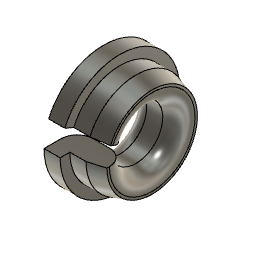
Cable Clamp (Autodesk Fusion 360 design; units mm, degrees)
Autodesk Fusion 360 part; units mm, degrees
note: some values were not read from the file. Set by a fixed rule: which sketch regions a step uses.
sketch "Sketch1" plane through (-35, 0, 0) normal (-1, 0, 0) x (0, -1, 0)
  circle A0 centre (-0.0027, 6.5006) radius 3
  spline S0 degree 3 poles (-2.3623, 9.8149) (-2.8292, 9.5488) (-3.2386, 9.1926) (-3.9138, 8.3291) (-4.1668, 7.8254) (-4.4751, 6.73) (-4.5197, 6.1469) (-4.3843, 4.9751) (-4.1979, 4.3986) (-3.7061, 3.5075) (-3.4567, 3.1707) (-2.8705, 2.5635) (-2.5345, 2.2973) (-2.1684, 2.078) knots 0 0 0 0 0.161221 0.161221 0.328565 0.328565 0.502029 0.502029 0.68161 0.68161 0.806401 0.806401 0.933976 0.933976 0.933976 0.933976
  arc A1 (-2.1684, 2.078) -> (2.1684, 2.078) centre (0, 6.5) ccw
  spline S1 degree 3 poles (2.1684, 2.078) (2.708, 2.4013) (3.1804, 2.8252) (3.9206, 3.816) (4.1875, 4.3686) (4.4856, 5.5258) (4.5215, 6.1173) (4.3635, 7.2597) (4.1789, 7.8006) (3.7084, 8.6093) (3.4817, 8.9033) (2.9632, 9.4172) (2.6753, 9.6365) (2.3623, 9.8149) knots 0 0 0 0 0.188714 0.188714 0.371292 0.371292 0.547732 0.547732 0.718032 0.718032 0.829274 0.829274 0.937741 0.937741 0.937741 0.937741
  arc A2 (2.3623, 9.8149) -> (-2.3623, 9.8149) centre (0, 6.5) ccw
  circle A3 centre (-0.0027, 6.5006) radius 3.7
  circle A4 centre (-0.0027, 6.5006) radius 3.1
  circle A5 centre (-0.0027, 6.5006) radius 1.65
  line L0 (-0.0027, 6.5006) -> (3.6973, 6.5006)
  line L1 (-0.0027, 6.5006) -> (3.4061, 7.9394)
  dimension "d1" = 7.4
  dimension "d2" = 3.3
  dimension "d3" = 6.2
  constraint concentric A0 A3
  constraint concentric A3 A4
  constraint concentric A3 A5
  constraint coincident A0.centre A3.centre
  constraint coincident A3 L0.end
  constraint horizontal L0
  constraint coincident A3 L1.end
  measures "d1" diameter of A3
  measures "d2" diameter of A5
  measures "d3" diameter of A4
extrude "Extrude1" add sketch "Sketch1" against normal blind 2 contours A0 A4 L0 L1 | A0 A5 L0 L1 picked at (-2.4687, 8.3112) picked at (2.5305, 6.2734)
extrude "Extrude2" add sketch "Sketch1" along normal blind 1 contours A0 A4 L0 | A0 A5 L0 L1 | A3 A4 L0 L1 picked at (2.295, 7.6295)
chamfer "Chamfer1" distance 0.3 distance2 1 1 edges at (-33, 3.0411, 5.8856) measured on face at (-33, -2.5968, 6.2685)
fillet "Fillet1" radius 1 1 edges at (-36, 1.6199, 6.1732)
fillet "Fillet2" radius 1 1 edges at (-33, 1.6199, 6.1732)
extrude "Extrude3" [suppressed]
extrude "Extrude4" [suppressed]
extrude "Extrude5" [suppressed]
named bodies: "Cable Clamp"
